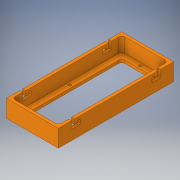
# Autodesk Inventor part: batteryholder
Saved by Autodesk Inventor 2017 (Build 210142000, 142)
## iProperties
Created: 2017-10-07
Part Number: batteryholder
Material: Generic
Document SubType Name: Modeling
Designer: User
Density: 1 g/cm^3
Appearance: Orange
Author: User
Autodesk Inventor part; units mm, degrees
ref_plane "YZ Plane" through (0, 0, 0) normal (1, 0, 0) x (0, 1, 0)
ref_plane "XZ Plane" through (0, 0, 0) normal (0, 1, 0) x (-1, 0, 0)
sketch "Sketch1" plane through (0, 0, 0) normal (0, 1, 0) x (-1, 0, 0)
  line L0 (0, 0) -> (3.175, 0)
  line L1 (3.175, 0) -> (3.175, -3.175)
  line L2 (3.175, -3.175) -> (0, -3.175)
  line L3 (0, -3.175) -> (0, 0)
  line L4 (0, 0) -> (6.35, 0)
  line L5 (0, -6.35) -> (0, 0)
  line L6 (3.175, 0) -> (50.8, 0)
  line L7 (50.8, 0) -> (50.8, -3.175)
  line L8 (50.8, -3.175) -> (3.175, -3.175)
  line L9 (3.175, -3.175) -> (3.175, 0)
  line L10 (50.8, 0) -> (57.15, 0)
  line L11 (57.15, 0) -> (57.15, -6.35)
  line L12 (57.15, 0) -> (53.975, 0)
  line L13 (53.975, 0) -> (53.975, -3.175)
  line L14 (53.975, -3.175) -> (57.15, -3.175)
  line L15 (57.15, -3.175) -> (57.15, 0)
  line L16 (53.975, -120.65) -> (53.975, -123.825)
  line L17 (53.975, -123.825) -> (50.8, -123.825)
  line L18 (57.15, -120.65) -> (57.15, -127)
  line L19 (57.15, -127) -> (50.8, -127)
  line L20 (3.175, -120.65) -> (3.175, -123.825)
  line L21 (3.175, -123.825) -> (6.35, -123.825)
  line L22 (0, -120.65) -> (0, -127)
  line L23 (0, -127) -> (6.35, -127)
  line L24 (53.975, -127) -> (57.15, -127)
  line L25 (57.15, -127) -> (57.15, 0)
  line L26 (57.15, 0) -> (53.975, 0)
  line L27 (53.975, 0) -> (53.975, -127)
  line L28 (50.8, -3.175) -> (57.15, -3.175)
  line L29 (57.15, -3.175) -> (57.15, 0)
  line L30 (57.15, 0) -> (50.8, 0)
  line L31 (50.8, 0) -> (50.8, -3.175)
  line L32 (50.8, -127) -> (6.35, -127)
  line L33 (6.35, -127) -> (6.35, -123.825)
  line L34 (6.35, -123.825) -> (50.8, -123.825)
  line L35 (50.8, -123.825) -> (50.8, -127)
  line L36 (0, -120.65) -> (3.175, -120.65)
  line L37 (3.175, -120.65) -> (3.175, -6.35)
  line L38 (3.175, -6.35) -> (0, -6.35)
  line L39 (0, -6.35) -> (0, -120.65)
  line L40 (3.175, -6.35) -> (3.175, -3.175)
  line L41 (3.175, -3.175) -> (6.35, -3.175)
  line L42 (53.975, -123.825) -> (57.15, -123.825)
  line L43 (57.15, -123.825) -> (57.15, -120.65)
  line L44 (57.15, -120.65) -> (53.975, -120.65)
  line L45 (53.975, -120.65) -> (53.975, -123.825)
  line L46 (0, -127) -> (3.175, -127)
  line L47 (3.175, -127) -> (3.175, -123.825)
  line L48 (3.175, -123.825) -> (0, -123.825)
  line L49 (0, -123.825) -> (0, -127)
  line L50 (3.175, -3.175) -> (6.35, -3.175)
  line L51 (6.35, -3.175) -> (6.35, 0)
  line L52 (6.35, 0) -> (3.175, 0)
  line L53 (3.175, 0) -> (3.175, -3.175)
  line L54 (57.15, -3.175) -> (53.975, -3.175)
  line L55 (53.975, -3.175) -> (53.975, -6.35)
  line L56 (53.975, -6.35) -> (57.15, -6.35)
  line L57 (57.15, -6.35) -> (57.15, -3.175)
  line L58 (57.15, -6.35) -> (53.975, -6.35)
  line L59 (53.975, -6.35) -> (53.975, -120.65)
  line L60 (53.975, -120.65) -> (57.15, -120.65)
  line L61 (57.15, -120.65) -> (57.15, -6.35)
  line L62 (3.175, -3.175) -> (0, -3.175)
  line L63 (0, -3.175) -> (0, -6.35)
  line L64 (0, -6.35) -> (3.175, -6.35)
  line L65 (3.175, -6.35) -> (3.175, -3.175)
  line L66 (3.175, -123.825) -> (0, -123.825)
  line L67 (0, -123.825) -> (0, -120.65)
  line L68 (0, -120.65) -> (3.175, -120.65)
  line L69 (3.175, -120.65) -> (3.175, -123.825)
  line L70 (3.175, -123.825) -> (6.35, -123.825)
  line L71 (6.35, -123.825) -> (6.35, -127)
  line L72 (6.35, -127) -> (3.175, -127)
  line L73 (3.175, -127) -> (3.175, -123.825)
  line L74 (53.975, -123.825) -> (50.8, -123.825)
  line L75 (50.8, -123.825) -> (50.8, -127)
  line L76 (50.8, -127) -> (53.975, -127)
  line L77 (53.975, -127) -> (53.975, -123.825)
  line L78 (57.15, -120.65) -> (53.975, -120.65)
  line L79 (53.975, -120.65) -> (53.975, -123.825)
  line L80 (53.975, -123.825) -> (57.15, -123.825)
  line L81 (57.15, -123.825) -> (57.15, -120.65)
  dimension "d2" = 3.175
  dimension "d3" = 3.175
  dimension "d7" = 6.35
  dimension "d8" = 3.175
  dimension "d9" = 3.175
  dimension "d10" = 3.175
  dimension "d11" = 3.175
  dimension "d12" = 6.35
  dimension "d13" = 6.35
  dimension "d14" = 3.175
  dimension "d15" = 3.175
  dimension "d16" = 6.35
  dimension "d17" = 6.35
  dimension "d18" = 3.175
  constraints: 164 end point, 34 parallel, 19 horizontal, 18 perpendicular, 1 midpoint, 1 point on line
  measures "d2" distance of L1.end L2.end
  measures "d3" distance of L0.end L1.end
  measures "d7" distance of L10.end L11.end
  measures "d8" distance of L14.end L13.end
  measures "d9" distance of L13.end L12.end
  measures "d10" distance of L16.end L17.end
  measures "d11" distance of L16.start L16.end
  measures "d12" distance of L18.end L19.end
  measures "d13" distance of L18.start L18.end
  measures "d14" distance of L21.end L20.end
  measures "d15" distance of L20.end L20.start
  measures "d16" distance of L23.end L22.end
  measures "d17" distance of L22.end L22.start
  measures "d18" distance of L52.end L4.end
extrude "Extrusion1" add sketch "Sketch1" along normal blind 19.05 contours L0 L1 L2 L3 | L4 L51 L8 L1 | L2 L40 L38 L5 | L6 L7 L8 L51 | L38 L37 L36 L39 | L10 L13 L28 L7 | L36 L20 L48 L22 | L10 L11 L14 L13 | L48 L47 L23 L22 | L14 L11 L56 L27 | L21 L33 L23 L47 | L56 L25 L44 L27 | L34 L35 L32 L33 | L44 L18 L42 L16 | L17 L27 L19 L35 | L42 L18 L19 L27
sketch "Sketch2" plane through (0, 0, 0) normal (0, -1, 0) x (1, 0, 0)
  line L0 (-3.175, -3.175) -> (-53.975, -3.175) projected
  line L1 (-53.975, -123.825) -> (-3.175, -123.825)
  line L2 (-3.175, -123.825) -> (-3.175, -3.175)
  line L3 (-3.175, -3.175) -> (-53.975, -3.175)
  line L4 (-53.975, -3.175) -> (-53.975, -123.825)
  line L5 (-53.975, -3.175) -> (-53.975, -123.825) projected
  line L6 (-53.975, -3.175) -> (-47.625, -3.175)
  line L7 (-47.625, -3.175) -> (-47.625, -9.525)
  line L8 (-47.625, -9.525) -> (-53.975, -9.525)
  line L9 (-53.975, -9.525) -> (-53.975, -3.175)
  line L10 (-3.175, -123.825) -> (-9.525, -123.825)
  line L11 (-9.525, -123.825) -> (-9.525, -117.475)
  line L12 (-9.525, -117.475) -> (-3.175, -117.475)
  line L13 (-3.175, -117.475) -> (-3.175, -123.825)
  line L14 (-47.625, -9.525) -> (-9.525, -9.525)
  line L15 (-9.525, -9.525) -> (-9.525, -117.475)
  line L16 (-9.525, -117.475) -> (-47.625, -117.475)
  line L17 (-47.625, -117.475) -> (-47.625, -9.525)
  point P0 (0, 0)
  dimension "d156" = 6.35
  dimension "d157" = 6.35
  dimension "d158" = 6.35
  dimension "d159" = 6.35
  constraints: 32 end point, 8 parallel, 4 horizontal, 4 perpendicular
  measures "d156" distance of L7.end L8.end
  measures "d157" distance between parallel lines of L0 L8
  measures "d158" distance of L11.end L12.end
  measures "d159" distance of L10.end L11.end
sketch "Sketch9" plane through (0, 0, 0) normal (1, 0, 0) x (0, 0, -1)
  line L0 (14.5789, 19.05) -> (17.7539, 19.05)
  line L1 (16.1664, 10.795) -> (16.1664, 10.795)
  line L2 (14.5789, 12.3825) -> (14.5789, 19.05)
  line L3 (16.1664, 10.795) -> (22.5164, 10.795)
  line L4 (20.9289, 13.97) -> (17.7539, 13.97)
  line L5 (24.1039, 12.3825) -> (24.1039, 14.9225)
  line L6 (20.9289, 14.9225) -> (20.9289, 13.97)
  line L7 (17.7539, 19.05) -> (17.7539, 13.97)
  line L8 (0, 0) -> (0, 19.05) projected
  line L9 (127, 0) -> (127, 19.05) projected
  line L10 (14.5789, 19.05) -> (17.7539, 19.05)
  line L11 (17.7539, 19.05) -> (17.7539, 13.97)
  line L12 (16.1664, 10.795) -> (14.5789, 10.795)
  line L13 (14.5789, 10.795) -> (14.5789, 19.05)
  line L14 (17.7539, 13.97) -> (20.9289, 13.97)
  line L15 (18.0714, 10.795) -> (16.1664, 10.795)
  line L16 (24.1039, 10.795) -> (18.0714, 10.795)
  line L17 (20.9289, 13.97) -> (20.9289, 16.51)
  line L18 (22.5164, 16.51) -> (22.5164, 16.51)
  line L19 (24.1039, 16.51) -> (24.1039, 10.795)
  line L20 (20.9289, 13.97) -> (17.7539, 13.97)
  line L21 (16.1664, 10.795) -> (18.0714, 10.795)
  line L22 (3.175, 19.05) -> (123.825, 19.05) projected
  line L23 (110.8336, 19.05) -> (112.4211, 19.05)
  line L24 (107.3411, 19.05) -> (108.9286, 19.05)
  line L25 (112.4211, 19.05) -> (110.8336, 19.05)
  line L26 (107.3411, 19.05) -> (108.9286, 19.05)
  line L27 (107.3411, 19.05) -> (108.9286, 19.05)
  line L28 (108.9286, 19.05) -> (110.8336, 19.05)
  line L29 (107.3411, 19.05) -> (108.9286, 19.05)
  line L30 (107.3411, 19.05) -> (108.9286, 19.05)
  line L31 (108.9286, 18.0911) -> (107.3411, 18.0911)
  line L32 (108.9286, 19.05) -> (110.8336, 19.05)
  line L33 (110.8336, 19.05) -> (112.4211, 19.05)
  line L34 (108.9286, 18.0911) -> (107.3411, 18.0911)
  line L35 (110.8336, 19.05) -> (112.4211, 19.05)
  line L36 (107.3411, 18.0911) -> (108.9286, 18.0911)
  line L37 (110.8336, 19.05) -> (108.9286, 19.05)
  line L38 (110.8336, 19.05) -> (112.4211, 19.05)
  line L39 (108.9286, 19.05) -> (110.8336, 19.05)
  line L40 (108.9286, 19.05) -> (110.8336, 19.05)
  line L41 (107.3411, 18.0911) -> (108.9286, 18.0911)
  line L42 (107.3411, 19.05) -> (108.9286, 19.05)
  line L43 (0, 19.05) -> (127, 19.05) projected
  arc A0 (14.5789, 12.3825) -> (16.1664, 10.795) centre (16.1664, 12.3825) ccw
  arc A1 (22.5164, 10.795) -> (24.1039, 12.3825) centre (22.5164, 12.3825) ccw
  arc A2 (24.1039, 14.9225) -> (22.5164, 16.51) centre (22.5164, 14.9225) ccw
  arc A3 (22.5164, 16.51) -> (20.9289, 14.9225) centre (22.5164, 14.9225) ccw
  dimension "d121" = 14.5789
  dimension "d190" = 3.175
  dimension "d191" = 3.175
  dimension "d192" = 3.175
  dimension "d193" = 3.175
  dimension "d194" = 2.54
  dimension "d195" = 2.54
  dimension "d196" = 1.5875
  dimension "d197" = 1.5875
  constraints: 80 end point, 18 horizontal, 10 parallel, 9 point on line, 8 point on circle, 8 tangent, 4 centre point, 2 equal radius, 2 perpendicular, 1 vertical
  measures "d121" distance between parallel lines of L2 L8
  measures "d190" distance between parallel lines of L19 L6
  measures "d191" distance between parallel lines of L2 L7
  measures "d192" distance between parallel lines of L3 L4
  measures "d193" distance between parallel lines of L17 L7
  measures "d194" distance between parallel lines of L4 L18
  measures "d195" distance between parallel lines of L18 L22
  measures "d196" radius of A0
  measures "d197" radius of A2
extrude "Extrusion9" cut sketch "Sketch9" against normal through all contours L0 L7 L4 L6 A3 A2 L5 A1 L3 A0 L2 | A0 L12 L13
extrude "Extrusion10" add sketch "Sketch2" against normal blind 3.175 contours L2 L12 L15 L14 L7 L0 | L7 L8 L4 L0 | L2 L1 L11 L12 | L17 L16 L11 L1 L4 L8
sketch "Sketch10" plane through (0, 3.175, 0) normal (0, 1, 0) x (1, 0, 0)
  circle A0 centre (-6.35, 63.5) radius 1.5875
  line L0 (-9.525, 117.475) -> (-9.525, 9.525) projected
  line L1 (-3.175, 123.825) -> (-3.175, 3.175) projected
  line L2 (-9.525, 9.525) -> (-47.625, 9.525) projected
  line L3 (-47.625, 9.525) -> (-47.625, 117.475) projected
  line L4 (-47.625, 117.475) -> (-9.525, 117.475) projected
  line L5 (-9.525, 117.475) -> (-9.525, 9.525) projected
  line L6 (-53.975, 123.825) -> (-3.175, 123.825) projected
  line L7 (-53.975, 3.175) -> (-53.975, 123.825) projected
  line L8 (-3.175, 3.175) -> (-53.975, 3.175) projected
  line L9 (-3.175, 123.825) -> (-3.175, 3.175) projected
  circle A1 centre (-50.8, 63.5) radius 1.5875
  circle A2 centre (-31.75, 6.35) radius 1.5875
  circle A3 centre (-30.1625, 120.65) radius 1.5875
  point P0 (0, 0)
  point P1 (-3.175, 110.8336)
  point P2 (-3.175, 17.7539)
  dimension "d163" = 3.175
  dimension "d166" = 3.175
  dimension "d167" = 120.65
  dimension "d168" = 60.325
  dimension "d169" = 3.175
  dimension "d170" = 1.5875
  dimension "d171" = 60.325
  dimension "d172" = 3.175
  dimension "d173" = 3.175
  dimension "d174" = 44.45
  dimension "d175" = 22.225
  dimension "d176" = 3.175
  dimension "d177" = 3.175
  dimension "d178" = 23.8125
  constraints: 4 centre point
  measures "d163" diameter of A0
  measures "d166" distance from line of A0.centre L0
  measures "d167" distance between parallel lines of L6 L8
  measures "d168" distance from line of L6 A0.centre
  measures "d169" diameter of A1
  measures "d170" distance edge to line of A1 L3
  measures "d171" distance from line of L6 A1.centre
  measures "d172" diameter of A2
  measures "d173" distance from line of L2 A2.centre
  measures "d174" distance between parallel lines of L0 L7
  measures "d175" distance from line of L7 A2.centre
  measures "d176" diameter of A3
  measures "d177" distance from line of L4 A3.centre
  measures "d178" distance from line of A3.centre L7
extrude "Extrusion11" cut sketch "Sketch10" against normal through all contours A0 | A1 | A2 | A3
fillet "Fillet1" radius 3.175 1 edges at (-53.975, 11.1125, -3.175)
fillet "Fillet2" radius 3.175 1 edges at (-53.975, 11.1125, -123.825)
fillet "Fillet3" radius 3.175 6 edges at (-3.175, 11.1125, -123.825) (-9.525, 1.5875, -117.475) (-3.175, 11.1125, -3.175) (-9.525, 1.5875, -9.525) (-47.625, 1.5875, -9.525) (-47.625, 1.5875, -117.475)
ref_plane "Work Plane1" through (-9.525, 3.175, -63.5) normal (0, 0, 1) x (1, 0, 0)
mirror "Mirror1" about plane through (-9.525, 3.175, -63.5) normal (0, 0, 1) of "Extrusion9"
ref_plane "Work Plane2" through (-9.525, 3.175, -63.5) normal (0, 0, 1) x (1, 0, 0)
body "Solid1"
